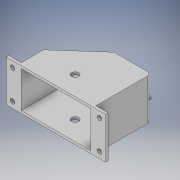
# Autodesk Inventor part: Radkasten_Links
Saved by Autodesk Inventor 2017 (Build 210142000, 142)
## iProperties
Part Number: Radkasten_Links
Material: Generisch
Document SubType Name: Modeling
Designer: Dima
Density: 1 g/cm^3
Appearance: Vorgabe
Author: Dima
Autodesk Inventor part; units mm, degrees
ref_plane "YZ Plane" through (0, 0, 0) normal (1, 0, 0) x (0, 1, 0)
ref_plane "XZ Plane" through (0, 0, 0) normal (0, 1, 0) x (-1, 0, 0)
ref_plane "XY Plane" through (0, 0, 0) normal (0, 0, 1) x (1, 0, 0)
sketch "Skizze1" plane through (0, 0, 0) normal (0, 1, 0) x (-1, 0, 0)
  line L0 (60, 25) -> (-60, 25)
  line L1 (-60, 25) -> (-60, -25)
  line L2 (-60, -25) -> (60, -25)
  line L3 (60, -25) -> (60, 25)
  point P0 (0, 0)
  point P1 (0, 25)
  point P2 (-60, 0)
  dimension "d0" = 120
  dimension "d1" = 50
  constraints: 8 end point, 2 midpoint, 2 parallel, 1 horizontal, 1 horizontal alignment, 1 perpendicular, 1 vertical alignment
  measures "d0" distance of L0.start L0.end
  measures "d1" distance of L2.end L0.start
extrude "Extrusion1" add sketch "Skizze1" along normal blind 70
sketch "Skizze2" plane through (60, 0, 25) normal (1, 0, 0) x (0, 0, -1)
  line L0 (0, 0) -> (50, 0) construction
  line L1 (50, 0) -> (50, 70) construction
  line L2 (0, 70) -> (50, 70) construction
  line L3 (0, 0) -> (0, 70) construction
  line L4 (0, 70) -> (50, 70)
  line L5 (50, 70) -> (50, 3)
  line L6 (50, 3) -> (0, 3)
  line L7 (0, 3) -> (0, 70)
  line L8 (50, 0) -> (50, 70) projected
  point P0 (25, 0)
  dimension "d4" = 3
  constraints: 8 end point, 2 parallel, 1 horizontal, 1 perpendicular, 1 point on line
  measures "d4" distance between parallel lines of L6 L0
extrude "Extrusion2" cut sketch "Skizze2" against normal blind 15
sketch "Skizze3" plane through (-60, 0, -25) normal (-1, 0, 0) x (0, 0, 1)
  line L0 (0, 0) -> (50, 0) construction
  line L1 (50, 0) -> (50, 70) construction
  line L2 (0, 70) -> (50, 70) construction
  line L3 (0, 0) -> (0, 70) construction
  line L4 (0, 70) -> (50, 70)
  line L5 (50, 70) -> (50, 3)
  line L6 (50, 3) -> (0, 3)
  line L7 (0, 3) -> (0, 70)
  line L8 (50, 0) -> (50, 70) projected
  point P0 (25, 0)
  dimension "d7" = 3
  constraints: 8 end point, 2 parallel, 1 horizontal, 1 perpendicular, 1 point on line
  measures "d7" distance between parallel lines of L0 L6
extrude "Extrusion3" cut sketch "Skizze3" against normal blind 15
shell "Wandung1" thickness 3 removed faces 1 at (20, 0, 8.3333)
sketch "Skizze4" plane through (0, 0, 0) normal (0, -1, 0) x (1, 0, 0)
  line L0 (42, 22) -> (42, -22) construction
  line L1 (42, -22) -> (-42, -22) construction
  line L2 (-42, -22) -> (-42, 22) construction
  line L3 (-42, 22) -> (42, 22) construction
  line L4 (-60, 25) -> (60, 25) construction
  line L5 (-60, -25) -> (-60, 25) construction
  line L6 (60, -25) -> (-60, -25) construction
  line L7 (60, 25) -> (60, -25) construction
  line L8 (-84, 0) -> (84, 0) construction
  line L9 (0, -35) -> (0, 35) construction
  point P0 (0, 0)
  point P1 (-52.5, -17.5)
  point P2 (-52.5, 17.5)
  point P3 (52.5, 17.5)
  point P4 (52.5, -17.5)
  dimension "d11" = 7.5
  dimension "d12" = 7.5
  constraints: 2 horizontal alignment, 2 symmetric about line, 2 vertical alignment
  measures "d11" distance from line of L5 point (-52.5, -17.5)
  measures "d12" distance from line of L4 point (-52.5, 17.5)
hole "Bohrung1" at (-52.5, 0, -17.5) at (-52.5, 0, 17.5) at (52.5, 0, 17.5) at (52.5, 0, -17.5) direction (0, 1, 0) diameter 5.5 end through all
sketch "Skizze5" plane through (60, 0, -25) normal (0, 0, -1) x (-1, 0, 0)
  line L0 (120, 3) -> (105, 3) projected
  line L1 (105, 3) -> (105, 70) projected
  line L2 (15, 70) -> (105, 70) projected
  line L3 (15, 70) -> (15, 3) projected
  line L4 (15, 3) -> (0, 3) projected
  line L5 (0, 0) -> (0, 3) projected
  line L6 (0, 0) -> (120, 0) projected
  line L7 (120, 0) -> (120, 3) projected
  point P0 (60, 0)
  point P1 (60, 23)
  point P2 (60, 0)
  dimension "d20" = 23
  constraints: 1 midpoint, 1 vertical alignment
  measures "d20" distance from line of L6 point (60, 23)
hole "Bohrung2" at (0, 23, -25) direction (0, 0, 1) diameter 8.5 end through all
sketch "Skizze6" plane through (-60, 0, 25) normal (0, 0, 1) x (1, 0, 0)
  circle A0 centre (60, 23) radius 4.25 construction
  line L0 (15, 3) -> (0, 3) construction
  line L1 (0, 0) -> (0, 3) construction
  line L2 (0, 0) -> (120, 0) construction
  line L3 (120, 0) -> (120, 3) construction
  line L4 (120, 3) -> (105, 3) construction
  line L5 (105, 3) -> (105, 70) construction
  line L6 (15, 70) -> (105, 70) construction
  line L7 (15, 70) -> (15, 3) construction
  line L8 (15, 70) -> (60, 70)
  line L9 (60, 70) -> (15, 30)
  line L10 (15, 30) -> (15, 70)
  line L11 (15, 70) -> (15, 3) projected
  point P0 (60, 0)
  dimension "d28" = 45
  dimension "d29" = 30
  constraints: 6 end point, 1 horizontal, 1 midpoint, 1 point on line
  measures "d28" distance of L6.start L8.end
  measures "d29" distance from line of L9.end L2
extrude "Extrusion4" cut sketch "Skizze6" against normal blind 25
sketch "Skizze7" plane through (0, 70, 0) normal (0, 1, 0) x (1, 0, 0)
  line L0 (0, 0) -> (0, -25) construction
  line L1 (0, -25) -> (45, -25) construction
  line L2 (45, -25) -> (45, 25) construction
  line L3 (45, 25) -> (-45, 25) construction
  line L4 (-45, 25) -> (-45, 0) construction
  line L5 (-45, 0) -> (0, 0) construction
  circle A0 centre (-10, 12.5) radius 3
  circle A1 centre (30, 12.5) radius 3
  point P0 (0, 0)
  point P1 (-45, 12.5)
  dimension "d32" = 6
  dimension "d34" = 6
  dimension "d35" = 40
  dimension "d43" = 15
  constraints: 2 centre point, 2 horizontal alignment, 1 midpoint
  measures "d32" diameter of A0
  measures "d34" diameter of A1
  measures "d35" distance of A1.centre A0.centre
  measures "d43" distance from line of L2 A1.centre
extrude "Extrusion5" add sketch "Skizze7" along normal blind 12
thread "Gewinde1" size "M6x1" class "6g" standard "ANSI Metric M Profile" full length
thread "Gewinde2" size "M6x1" class "6g" standard "ANSI Metric M Profile" full length
fillet "Rundung1" radius 5 4 edges at (42, 67, 0) (-42, 67, -11) (-45, 70, -12.5) (45, 70, 0)
equation "\"d12\" = d11"
